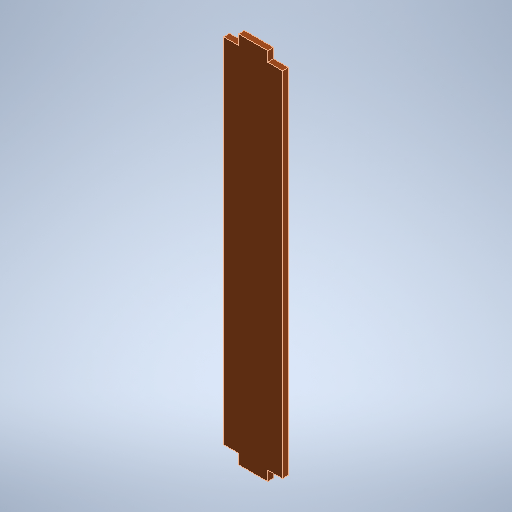
# Autodesk Inventor part: Assembly Fixation Rod
Saved by Autodesk Inventor 2025.4 (Build 294407000, 407)
## iProperties
Created: 2026-05-09
Part Number: Assembly Fixation Rod
Material: Generic
Document SubType Name: Sheet Metal
Designer: lenovo
Density: 1 g/cm^3
Sheet Metal Rule: Default_mm
Appearance: Default(1)
Author: lenovo
Autodesk Inventor part; units mm, degrees
ref_plane "YZ Plane" through (0, 0, 0) normal (1, 0, 0) x (0, 1, 0)
ref_plane "XZ Plane" through (0, 0, 0) normal (0, 1, 0) x (-1, 0, 0)
ref_plane "XY Plane" through (0, 0, 0) normal (0, 0, 1) x (1, 0, 0)
sketch "Sketch1" plane through (0, 0, 0) normal (0, 0, 1) x (1, 0, 0)
  line L0 (-15, -90) -> (15, -90)
  line L1 (15, -90) -> (15, 90)
  line L2 (15, 90) -> (-15, 90)
  line L3 (-15, 90) -> (-15, -90)
  line L4 (-15, -90) -> (15, 90) construction
  line L5 (15, -90) -> (-15, 90) construction
  line L6 (-7.45, 95.1) -> (7.45, 95.1)
  line L7 (7.45, 95.1) -> (7.45, 90)
  line L8 (7.45, 90) -> (-7.45, 90)
  line L9 (-7.45, 90) -> (-7.45, 95.1)
  line L10 (-7.45, 95.1) -> (7.45, 90) construction
  line L11 (7.45, 95.1) -> (-7.45, 90) construction
  line L12 (-15, 0) -> (15, 0)
  line L13 (-7.45, -95.1) -> (7.45, -95.1)
  line L14 (7.45, -95.1) -> (7.45, -90)
  line L15 (7.45, -90) -> (-7.45, -90)
  line L16 (-7.45, -90) -> (-7.45, -95.1)
  line L17 (-7.45, -95.1) -> (7.45, -90) construction
  line L18 (7.45, -95.1) -> (-7.45, -90) construction
  point P0 (0, 0)
  point P1 (0, 92.55)
  point P2 (0, 90)
  point P3 (0, -90)
  dimension "d0" = 180
  dimension "d1" = 30
  dimension "d2" = 14.9
  dimension "d3" = 5.1
  measures "d0" distance of L1.end L0.end
  measures "d1" distance between parallel lines of L3 L1
  measures "d2" distance of L6.start L6.end
  measures "d3" distance of L6.end L7.end
extrude "Plate1" add sketch "Sketch1" along normal blind 3
equation "\"d4\" = Thickness"
equation "\"BendRadius\" = Thickness"
equation "\"BendReliefWidth\" = Thickness"
equation "\"BendReliefDepth\" = 0.5 * Thickness"
equation "\"CornerReliefSize\" = 4 * Thickness"
equation "\"MinimumRemnant\" = 2 * Thickness"
equation "\"TransitionRadius\" = BendRadius"
equation "\"JacobiRadiusSize\" = BendRadius"
equation "\"GapSize\" = Thickness"
equation "\"Thickness\" = 3"
body "Solid1"
